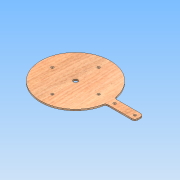
# Autodesk Inventor part: Top_Lever Side
Saved by Autodesk Inventor 2018.1 (Build 221171000, 171)
## iProperties
Created: 2019-03-23
Part Number: Top_Lever Side
Material: Wood (Birch)
Document SubType Name: Modeling
Designer: James
Density: 0.55 g/cm^3
Appearance: Birch - Natural Polished
Author: James
Autodesk Inventor part; units mm, degrees
ref_plane "YZ Plane" through (0, 0, 0) normal (1, 0, 0) x (0, 1, 0)
ref_plane "XZ Plane" through (0, 0, 0) normal (0, 1, 0) x (-1, 0, 0)
ref_plane "XY Plane" through (0, 0, 0) normal (0, 0, 1) x (1, 0, 0)
sketch "Sketch1" plane through (0, 0, 0) normal (0, 0, 1) x (1, 0, 0)
  circle A0 centre (0, 0) radius 120
  line L0 (100, 15) -> (220, 15)
  line L1 (220, 15) -> (220, -15)
  line L2 (220, -15) -> (100, -15)
  line L3 (100, -15) -> (100, 15)
  dimension "d0" = 240
  dimension "d1" = 30
  dimension "d2" = 15
  dimension "d3" = 100
  dimension "d4" = 220
  constraints: 8 end point, 2 parallel, 1 centre point, 1 coincident, 1 horizontal, 1 perpendicular
  measures "d0" diameter of A0
  measures "d1" distance between parallel lines of L2 L0
  measures "d2" distance from line of point (0, 0) L0
  measures "d3" distance from line of point (0, 0) L3
  measures "d4" distance from line of point (0, 0) L1
extrude "Extrusion1" add sketch "Sketch1" along normal blind 5
fillet "Fillet1" radius 10 4 edges at (119.0588, -15, 2.5) (119.0588, 15, 2.5) (220, -15, 2.5) (220, 15, 2.5)
sketch "Sketch2" plane through (0, 0, 5) normal (0, 0, 1) x (1, 0, 0)
  line L0 (220, -5) -> (220, 5) projected
  point P0 (0, 0)
  point P1 (135, 0)
  point P2 (205, 0)
  point P3 (220, 0)
  dimension "d8" = 15
  dimension "d9" = 70
  constraints: 2 horizontal alignment, 1 midpoint
  measures "d8" distance from line of point (205, 0) L0
  measures "d9" distance of point (205, 0) point (135, 0)
hole "Hole1" at (135, 0, 5) at (205, 0, 5) direction (0, 0, -1) diameter 4.496 end through all countersink diameter 8.433 countersink angle 82 clearance for "Flat Head Machine Screw (82)" size "#8" standard "Ansi Unified Screw Threads"
sketch "Sketch3" plane through (0, 0, 5) normal (0, 0, 1) x (1, 0, 0)
  point P0 (0, 0)
  point P1 (0, 80)
  dimension "d17" = 80
  constraints: 1 vertical alignment
  measures "d17" distance of point (0, 0) point (0, 80)
hole "Hole2" at (0, 80, 5) direction (0, 0, -1) diameter 4.496 end through all countersink diameter 8.433 countersink angle 82 clearance for "Flat Head Machine Screw (82)" size "#8" standard "Ansi Unified Screw Threads"
pattern_circular "Circular Pattern1" count 4 over 360 about axis through (0, 0, -10) along (0, 0, 1) of "Hole2"
sketch "Sketch4" plane through (0, 0, 5) normal (0, 0, 1) x (1, 0, 0)
  point P0 (0, 0)
  point P1 (0, 0)
  constraints: 1 coincident
hole "Hole3" at (0, 0, 5) direction (0, 0, -1) diameter 15 end through all
equation "\"d2\" = 0.5 * d1"
body "Solid1"
